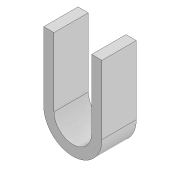
# Autodesk Inventor part: Plate_clip
Saved by Autodesk Inventor 2022 (Build 260153000, 153)
## iProperties
Created: 2022-07-29
Part Number: Plate_clip
Material: Generic
Document SubType Name: Modeling
Designer: dell
Density: 1 g/cm^3
Appearance: Default
Author: dell
Autodesk Inventor part; units mm, degrees
ref_plane "YZ Plane" through (0, 0, 0) normal (1, 0, 0) x (0, 1, 0)
ref_plane "XZ Plane" through (0, 0, 0) normal (0, 1, 0) x (-1, 0, 0)
ref_plane "XY Plane" through (0, 0, 0) normal (0, 0, 1) x (1, 0, 0)
sketch "Sketch1" plane through (0, 0, 0) normal (0, 0, 1) x (1, 0, 0)
  line L0 (-8.5, 0) -> (-5.5, 0)
  line L1 (-5.5, 0) -> (-5.5, 20)
  line L2 (-5.5, 20) -> (-8.5, 20)
  line L3 (-8.5, 20) -> (-8.5, 0)
  line L4 (8.5, 0) -> (5.5, 0)
  line L5 (5.5, 0) -> (5.5, 20)
  line L6 (5.5, 20) -> (8.5, 20)
  line L7 (8.5, 20) -> (8.5, 0)
  arc A0 (-5.5, 0) -> (5.5, 0) centre (0, 0) ccw
  arc A1 (-8.5, 0) -> (8.5, 0) centre (0, 0) ccw
  point P0 (0, 0)
  dimension "d0" = 3
  dimension "d1" = 3
  dimension "d2" = 5.5
  dimension "d3" = 5.5
  dimension "d4" = 20
  dimension "d5" = 20
  constraints: 16 end point, 4 parallel, 4 point on circle, 4 tangent, 2 centre point, 2 horizontal, 2 perpendicular, 2 point on line
  measures "d0" distance between parallel lines of L3 L1
  measures "d1" distance between parallel lines of L7 L5
  measures "d2" distance from line of point (0, 0) L1
  measures "d3" distance from line of point (0, 0) L5
  measures "d4" distance between parallel lines of L0 L2
  measures "d5" distance between parallel lines of L4 L6
extrude "Extrusion1" add sketch "Sketch1" along normal blind 10
body "Solid1"
